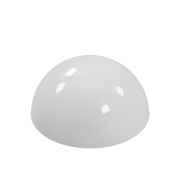
# Autodesk Inventor part: 11_Range
Saved by Autodesk Inventor 2022 (Build 260153000, 153)
## iProperties
Created: 2022-06-10
Part Number: 11_Range
Material: Generic
Document SubType Name: Modeling
Designer: pzach
Density: 1 g/cm^3
Appearance: Sky Blue Medium
Author: pzach
Autodesk Inventor part; units mm, degrees
ref_plane "YZ Plane" through (0, 0, 0) normal (1, 0, 0) x (0, 1, 0)
ref_plane "XZ Plane" through (0, 0, 0) normal (0, 1, 0) x (-1, 0, 0)
ref_plane "XY Plane" through (0, 0, 0) normal (0, 0, 1) x (1, 0, 0)
sketch "Sketch2" plane through (0, 0, 0) normal (1, 0, 0) x (0, 1, 0)
  arc A0 (0, -6000) -> (0, 6000) centre (0, 0) ccw
  line L0 (0, -6000) -> (0, 6000)
  dimension "d2" = 12000
  dimension "d3" = 12000
  constraints: 2 end point, 2 point on circle, 1 centre point, 1 coincident, 1 vertical
  measures "d2" diameter of A0
  measures "d3" distance of L0.start L0.end
extrude "Extrusion1" add sketch "Sketch2" along normal mid plane 12000
fillet "Fillet1" radius 6000 2 edges at (6000, 6000, 0) (-6000, 6000, 0)
equation "\"d3\" = d2"
equation "\"d4\" = d2"
equation "\"d6\" = 0.5 * d2"
body "Solid1"
